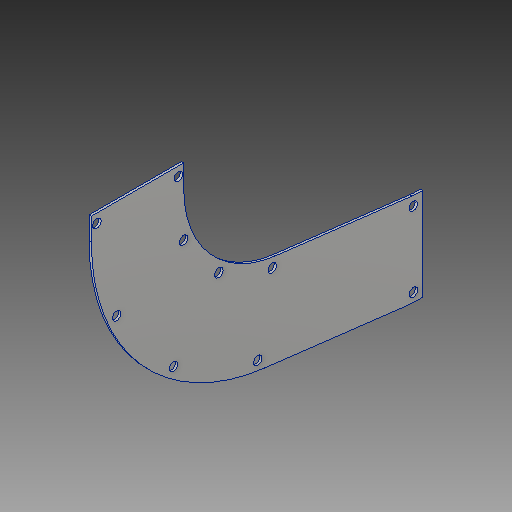
# Autodesk Inventor part: Storage Side Plate
Saved by Autodesk Inventor 2019.4 (Build 234330000, 330)
## iProperties
Created: 2020-01-11
Part Number: Storage Side Plate
Material: Aluminum 6061
Document SubType Name: Modeling
Designer: admin
Density: 2.7 g/cm^3
Appearance: Aluminum - Flat
Author: admin
Autodesk Inventor part; units mm, degrees
ref_plane "YZ Plane" through (0, 0, 0) normal (1, 0, 0) x (0, 1, 0)
ref_plane "XZ Plane" through (0, 0, 0) normal (0, 1, 0) x (-1, 0, 0)
ref_plane "XY Plane" through (0, 0, 0) normal (0, 0, 1) x (1, 0, 0)
sketch "Sketch1" plane through (0, 0, 0) normal (1, 0, 0) x (0, 1, 0)
  arc A0 (273.7291, -166.7427) -> (45.384, -369.2015) centre (273.7291, -396.7427) ccw
  arc A1 (273.7291, 36.4573) -> (-156.3539, -344.8694) centre (273.7291, -396.7427) ccw
  line L0 (45.384, -369.2015) -> (9.2003, -669.2015)
  line L1 (-156.3539, -344.8694) -> (-192.5376, -644.8694)
  line L2 (48.9453, -381.4304) -> (48.9453, -441.4304) projected
  line L3 (-161.2547, -373.9304) -> (-161.2547, -293.9304) projected
  arc A2 (9.2003, -669.2015) -> (7.7612, -693.1504) centre (207.7612, -693.1504) ccw
  arc A3 (-192.5376, -644.8694) -> (-195.4388, -693.1504) centre (207.7612, -693.1504) ccw
  line L4 (-195.4388, -693.1504) -> (7.7612, -693.1504)
  line L5 (48.9453, -381.4304) -> (21.7149, -607.1979) construction
  line L6 (-161.2547, -373.9304) -> (-171.9549, -462.646) construction
  line L7 (273.7291, 36.4573) -> (323.7291, 36.4573)
  line L8 (323.7291, 36.4573) -> (323.7291, -166.7427)
  line L9 (323.7291, -166.7427) -> (273.7291, -166.7427)
  dimension "d4" = 203.2
  dimension "d6" = 5
  dimension "d7" = 1.3856
  dimension "d8" = 230
  dimension "d9" = 300
  dimension "d10" = 200
  dimension "d35" = 50
  constraints: 16 end point, 8 point on circle, 5 tangent, 4 centre point, 4 parallel, 2 coincident, 2 horizontal, 2 perpendicular, 1 line through centre
  measures "d4" distance of L7.start L9.end
  measures "d6" distance between parallel lines of L5 L0
  measures "d7" distance between parallel lines of L1 L6
  measures "d8" radius of A0
  measures "d9" vertical distance of L0.start L0.end
  measures "d10" radius of A2
  measures "d35" distance of L7.start L7.end
extrude "Extrusion1" add sketch "Sketch1" along normal blind 5
sketch "Sketch2" plane through (5, 0, 0) normal (1, 0, 0) x (0, 0, -1)
  line L0 (671.8238, -11.261) -> (361.5723, 26.1592) construction
  line L1 (361.5723, 26.1592) -> (244.1052, 75.7347) construction
  line L2 (244.1052, 75.7347) -> (166.3168, 176.7555) construction
  line L3 (166.3168, 176.7555) -> (154.7427, 303.7291) construction
  circle A0 centre (671.8238, -11.261) radius 9.5
  circle A1 centre (361.5723, 26.1592) radius 9.5
  circle A2 centre (244.1052, 75.7347) radius 9.5
  circle A3 centre (166.3168, 176.7555) radius 9.5
  circle A4 centre (154.7427, 303.7291) radius 9.5
  line L4 (669.2015, 9.2003) -> (369.2015, 45.384) construction
  circle A5 centre (72.4572, -74.3053) radius 88.9 construction
  line L5 (244.1052, 75.7347) -> (256.3162, 91.5742) construction
  arc A6 (166.7427, 273.7291) -> (369.2015, 45.384) centre (396.7427, 273.7291) ccw construction
  line L6 (166.3168, 176.7555) -> (184.7508, 184.5134) construction
  line L7 (672.2554, -175.6958) -> (329.7378, -134.3839) construction
  line L8 (329.7378, -134.3839) -> (144.1809, -53.2981) construction
  line L9 (144.1809, -53.2981) -> (19.128, 105.9753) construction
  line L10 (19.128, 105.9753) -> (-24.4573, 303.7291) construction
  circle A7 centre (672.2554, -175.6958) radius 9.5
  circle A8 centre (329.7378, -134.3839) radius 9.5
  circle A9 centre (144.1809, -53.2981) radius 9.5
  circle A10 centre (19.128, 105.9753) radius 9.5
  circle A11 centre (-24.4573, 303.7291) radius 9.5
  line L11 (-24.4573, 303.7291) -> (154.7427, 303.7291) construction
  line L12 (344.8694, -156.3539) -> (644.8694, -192.5376) projected
  circle A12 centre (154.7427, 303.7291) radius 25.4 construction
  circle A13 centre (-24.4573, 303.7291) radius 25.4 construction
  line L13 (19.128, 105.9753) -> (0.8504, 97.8555) construction
  arc A14 (-36.4573, 273.7291) -> (344.8694, -156.3539) centre (396.7427, 273.7291) ccw projected
  line L14 (166.7427, 323.7291) -> (-36.4573, 323.7291) projected
  line L15 (693.1504, -195.4388) -> (693.1504, 7.7612) projected
  line L16 (144.1809, -53.2981) -> (131.9563, -69.1271) construction
  point P0 (0, 0)
  dimension "d11" = 312.5
  dimension "d12" = 19
  dimension "d13" = 19
  dimension "d14" = 19
  dimension "d15" = 19
  dimension "d16" = 19
  dimension "d18" = 12
  dimension "d19" = 20
  dimension "d20" = 177.8
  dimension "d21" = 20
  dimension "d22" = 20
  dimension "d23" = 19
  dimension "d24" = 19
  dimension "d25" = 19
  dimension "d26" = 19
  dimension "d28" = 19
  dimension "d29" = 20
  dimension "d30" = 50.8
  dimension "d31" = 50.8
  dimension "d34" = 20
  dimension "d36" = 20
  dimension "d37" = 20.895
  dimension "d38" = 20
  dimension "d39" = 202.5
  dimension "d40" = 127.5
  dimension "d41" = 345
  dimension "d42" = 202.5
  dimension "d43" = 202.5
  dimension "d44" = 127.5
  dimension "d46" = 127.5
  dimension "d49" = 12
  constraints: 26 end point, 13 centre point, 11 coincident, 4 line through centre, 4 point on circle, 1 horizontal, 1 parallel
  measures "d11" distance of L0.start L0.end
  measures "d12" diameter of A0
  measures "d13" diameter of A1
  measures "d14" diameter of A2
  measures "d15" diameter of A3
  measures "d16" diameter of A4
  measures "d18" horizontal distance of A6.start L11.end
  measures "d19" distance from line of L4 A1.centre
  measures "d20" diameter of A5
  measures "d21" distance of L5.start L5.end
  measures "d22" distance of L6.start L6.end
  measures "d23" diameter of A7
  measures "d24" diameter of A8
  measures "d25" diameter of A9
  measures "d26" diameter of A10
  measures "d28" diameter of A11
  measures "d29" distance between parallel lines of L12 L7
  measures "d30" diameter of A12
  measures "d31" diameter of A13
  measures "d34" distance of L13.start L13.end
  measures "d36" distance from line of L14 L11.end
  measures "d37" distance from line of L15 L7.start
  measures "d38" distance of L16.start L16.end
  measures "d39" distance of L7.end L8.end
  measures "d40" distance of L0.end L1.end
  measures "d41" distance of L7.start L7.end
  measures "d42" distance of L8.end L9.end
  measures "d43" distance of L10.end L9.end
  measures "d44" distance of L1.end L2.end
  measures "d46" distance of L2.end L3.end
  measures "d49" horizontal distance of L14.end L10.end
extrude "Extrusion2" cut sketch "Sketch2" against normal through all
body "Solid1"
